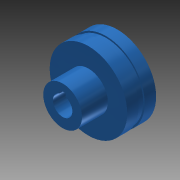
# Autodesk Inventor part: Puller Wheel
Saved by Autodesk Inventor 2014 SP1 (Build 180222100, 222)
## iProperties
Created: 2014-11-17
Part Number: Puller Wheel
Material: Generic
Document SubType Name: Modeling
Designer: AlecShufelt
Density: 1 g/cm^3
Appearance: Cyan
Author: AlecShufelt
Autodesk Inventor part; units mm, degrees
ref_plane "YZ Plane" through (0, 0, 0) normal (1, 0, 0) x (0, 1, 0)
ref_plane "XZ Plane" through (0, 0, 0) normal (0, 1, 0) x (-1, 0, 0)
ref_plane "XY Plane" through (0, 0, 0) normal (0, 0, 1) x (1, 0, 0)
sketch "Sketch4" plane through (0, 0, 0) normal (0, 0, 1) x (1, 0, 0)
  circle A0 centre (0, 0) radius 18.3
  dimension "d9" = 36.6
  constraints: 1 centre point, 1 coincident
  measures "d9" diameter of A0
extrude "Extrusion4" add sketch "Sketch4" along normal blind 3
sketch "Sketch5" plane through (0, 0, 3) normal (0, 0, 1) x (1, 0, 0)
  circle A0 centre (0, 0) radius 18.3 projected
  circle A1 centre (0, 0) radius 19.05
  dimension "d12" = 38.1
  constraints: 1 centre point, 1 coincident
  measures "d12" diameter of A1
extrude "Extrusion5" add sketch "Sketch5" along normal blind 5.6 contours A0 | A1
sketch "Sketch6" plane through (0, 0, 0) normal (0, 0, -1) x (-1, 0, 0)
  circle A0 centre (0, 0) radius 18.3 projected
  circle A1 centre (0, 0) radius 19.05
  dimension "d15" = 38.1
  constraints: 1 centre point, 1 coincident
  measures "d15" diameter of A1
extrude "Extrusion6" add sketch "Sketch6" along normal blind 5.6 contours A0 | A1
sketch "Sketch7" plane through (0, 0, 8.6) normal (0, 0, 1) x (1, 0, 0)
  circle A0 centre (0, 0) radius 19.05 projected
  circle A1 centre (0, 0) radius 9.525
  dimension "d18" = 19.05
  constraints: 1 centre point, 1 coincident
  measures "d18" diameter of A1
extrude "Extrusion7" add sketch "Sketch7" along normal blind 12.7 contours A1
sketch "Sketch8" plane through (0, 0, -5.6) normal (0, 0, -1) x (-1, 0, 0)
  circle A0 centre (0, 0) radius 19.05 projected
  circle A1 centre (0, 0) radius 4.7625
  dimension "d21" = 9.525
  constraints: 1 centre point, 1 coincident
  measures "d21" diameter of A1
extrude "Extrusion8" cut sketch "Sketch8" against normal blind 38.1 contours A1
sketch "Sketch9" plane through (0, 0, -5.6) normal (0, 0, -1) x (-1, 0, 0)
  circle A0 centre (0, 0) radius 4.7625 projected
  line L0 (-1.4638, 3.2131) -> (1.4638, 3.2131)
  line L1 (1.4638, 3.2131) -> (1.4638, 6.1406)
  line L2 (1.4638, 6.1406) -> (-1.4638, 6.1406)
  line L3 (-1.4638, 6.1406) -> (-1.4638, 3.2131)
  dimension "d24" = 2.9276
  dimension "d25" = 2.9276
  dimension "d26" = 3.2131
  dimension "d27" = 1.4638
  constraints: 8 end point, 2 parallel, 1 horizontal, 1 perpendicular
  measures "d24" distance between parallel lines of L2 L0
  measures "d25" distance between parallel lines of L3 L1
  measures "d26" distance from line of L0 A0.centre
  measures "d27" distance from line of A0.centre L3
extrude "Extrusion9" cut sketch "Sketch9" against normal blind 38.1 contours L1 L0 L3 A0 | A0 L3 L2 L1 picked at (0.165, 3.721)
equation "\"d25\" = d24"
equation "\"d27\" = 0.5 * d25"
body "Solid2"
